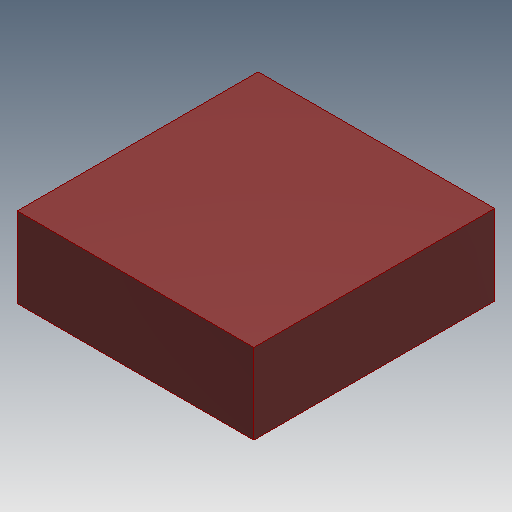
# Autodesk Inventor part: 3_3V
Saved by Autodesk Inventor 2017 (Build 210142000, 142)
## iProperties
Part Number: 3_3V
Material: Generisch
Document SubType Name: Modeling
Designer: Werkstatt
Density: 1 g/cm^3
Appearance: SOT23-5, 3_3V
Author: Werkstatt
Autodesk Inventor part; units mm, degrees
ref_plane "YZ Plane" through (0, 0, 0) normal (1, 0, 0) x (0, 1, 0)
ref_plane "XZ Plane" through (0, 0, 0) normal (0, 1, 0) x (-1, 0, 0)
ref_plane "XY Plane" through (0, 0, 0) normal (0, 0, 1) x (1, 0, 0)
sketch "SOT23-5, 3_3V_64" plane through (0, 0, 0) normal (0, 0, 1) x (1, 0, 0)
  line L0 (-1.4224, 1.5) -> (1.524, 1.5)
  line L1 (1.524, 1.5) -> (1.524, -1.5)
  line L2 (1.524, -1.5) -> (-1.4224, -1.5)
  line L3 (-1.4224, -1.5) -> (-1.4224, 1.5)
  constraints: 8 end point
extrude "Extrusion1" add sketch "SOT23-5, 3_3V_64" along normal blind 1
